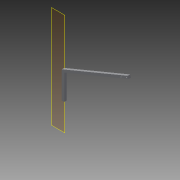
# Autodesk Inventor part: Catapult
Saved by Autodesk Inventor 2013 (Build 170138000, 138)
## iProperties
Created: 2014-01-16
Part Number: Catapult
Material: Generic
Document SubType Name: Modeling
Designer: 215152
Density: 1 g/cm^3
Author: 215152
Autodesk Inventor part; units mm, degrees
ref_plane "YZ Plane" through (0, 0, 0) normal (1, 0, 0) x (0, 1, 0)
ref_plane "XZ Plane" through (0, 0, 0) normal (0, 1, 0) x (-1, 0, 0)
ref_plane "XY Plane" through (0, 0, 0) normal (0, 0, 1) x (1, 0, 0)
ref_plane "Work Plane1" through (0, -120.8432, 0) normal (0, 0, 1) x (1, 0, 0)
sketch "Sketch1" plane through (0, -120.8432, 0) normal (0, 0, 1) x (1, 0, 0)
  line L0 (0, 120.8432) -> (63.5, 120.8432)
  line L1 (63.5, 120.8432) -> (63.5, 603.4432)
  line L2 (63.5, 603.4432) -> (0, 603.4432)
  line L3 (0, 603.4432) -> (0, 120.8432)
  line L4 (63.5, 603.4432) -> (-63.5, 603.4432)
  line L5 (-63.5, 603.4432) -> (-63.5, 527.2432)
  line L6 (-63.5, 527.2432) -> (63.5, 527.2432)
  line L7 (63.5, 527.2432) -> (63.5, 603.4432)
  line L8 (63.5, 527.2432) -> (63.5, 349.4432)
  line L9 (63.5, 527.2432) -> (241.3, 527.2432) construction
  line L10 (63.5, 527.2432) -> (1409.7, 527.2432)
  line L11 (1409.7, 527.2432) -> (1409.7, 349.4432)
  line L12 (1409.7, 349.4432) -> (63.5, 349.4432)
  line L13 (63.5, 349.4432) -> (63.5, 527.2432)
  line L14 (1409.7, 438.3432) -> (63.5, 438.3432)
  line L15 (736.6, 438.3432) -> (736.6, 349.4432)
  circle A0 centre (736.6, 438.3432) radius 88.9
  line L16 (736.6, 438.3432) -> (800.1, 438.3432) construction
  circle A1 centre (677.9336, 293.1996) radius 6.35
  circle A2 centre (736.6, 438.3432) radius 6.35
  line L17 (736.6, 438.3432) -> (1465.1582, 438.3432) construction
  line L18 (736.6, 438.3432) -> (754.1999, 445.6333)
  line L19 (736.6, 438.3432) -> (755.65, 438.3432) construction
  line L20 (754.1999, 445.6333) -> (759.06, 433.9)
  line L21 (759.06, 433.9) -> (749.3398, 457.3666)
  line L22 (749.3398, 457.3666) -> (63.5, 173.2824)
  line L23 (759.06, 433.9) -> (63.5, 145.7896)
  line L24 (759.06, 433.9) -> (1511.9287, 433.9) construction
  line L25 (63.5, 145.7896) -> (63.5, -108.2104)
  line L26 (63.5, -108.2104) -> (38.1, -108.2104)
  line L27 (63.5, -108.2104) -> (88.9, -108.2104)
  line L28 (63.5, -108.2104) -> (88.9, -108.2104) construction
  line L29 (88.9, -108.2104) -> (88.9, 156.3107)
  dimension "d0" = 63.5
  dimension "d1" = 482.6
  dimension "d2" = 127
  dimension "d3" = 76.2
  dimension "d4" = 177.8
  dimension "d5" = 90
  dimension "d6" = 1346.2
  dimension "d7" = 177.8
  dimension "d10" = 12.7
  dimension "d11" = 12.7
  dimension "d13" = 19.05
  dimension "d14" = 22.5
  dimension "d15" = 12.7
  dimension "d16" = 25.4
  dimension "d17" = 90
  dimension "d18" = 157.5
  dimension "d19" = 254
  dimension "d20" = 25.4
  dimension "d21" = 90
  dimension "d22" = 25.4
  dimension "d23" = 0
  constraints: 60 end point, 9 horizontal, 8 perpendicular, 6 parallel, 4 equal length, 4 midpoint, 3 point on line, 2 centre point, 2 coincident, 1 collinear, 1 vertical alignment, 2 other
  measures "d0" distance of L2.end L1.end
  measures "d1" distance of L1.end L0.end
  measures "d2" distance of L6.end L5.end
  measures "d3" distance of L5.end L4.end
  measures "d4" distance of L6.end L8.end
  measures "d5" angle of L8 L9
  measures "d6" distance of L11.end L12.end
  measures "d7" distance of L10.end L11.end
  measures "d10" diameter of A1
  measures "d11" diameter of A2
  measures "d13" distance of L17.start L18.end
  measures "d14" angle of L19 L18
  measures "d15" distance of L18.end L20.end
  measures "d16" distance of L20.end L21.end
  measures "d17" angle of L22 L21
  measures "d18" angle of L23 L24
  measures "d19" distance of L23.end L25.end
  measures "d20" distance of L25.end L26.end
  measures "d21" angle of L25 L26
  measures "d22" distance of L25.end L27.end
  measures "d23" distance between parallel lines of L27 L28
extrude "Extrusion1" add sketch "Sketch1" along normal blind 25.4 contours L1 L23 L29 L27 L25 | L1 L22 L12 L23 | L22 A0 L23 L12 | L22 L14 A2 L15 L23 A0 | L22 L21 L18 A2 L14 | L20 L23 L15 A2 L14 | L14 A2 L18 L20
body "Solid1"
